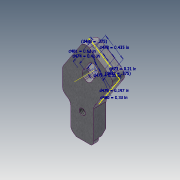
# Autodesk Inventor part: J005520
Saved by Autodesk Inventor 2015 SP1 (Build 190203100, 203)
## iProperties
Created: 2014-10-30
Material: STAINLESS STEEL, 303
Vendor: HHMI: JFRC - ID&F
Document SubType Name: Modeling
Designer: arnoldj
Density: 8 g/cm^3
Mass: 37.2011 g
Surface Area: 34.3864 cm^2
Volume: 4.65014 cm^3
Description: MBS TRAINER CLAMP ARM
Project: P-201804
Appearance: Metal-Steel (Stainless, Brushed)
Part Number: J005520
RuleStatus: InUse
AfterDocSave0: file://Part Number Cleaner
LAB/DEPT: SVOBODA (LAB)
REQUESTING SCIENTIST: SOFRONIEW, NICK
SURFACE ROUGHNESS: 63 Ra
DESIGN DEPARTMENT: HHMI: JRC - ID&F
SPECIAL FINISH: NONE
ALTERED ITEM PART NUMBER: N/A
ALTERED ITEM VENDOR: N/A
ALTERED ITEM DESCRIPTION: N/A
Revision Number: -
Autodesk Inventor part; units mm, degrees
ref_plane "YZ Plane" through (0, 0, 0) normal (1, 0, 0) x (0, 1, 0)
ref_plane "XZ Plane" through (0, 0, 0) normal (0, 1, 0) x (-1, 0, 0)
sketch "Sketch1" plane through (0, 0, 0) normal (0, 0, 1) x (1, 0, 0)
  line L0 (-6, 18.161) -> (6, 18.161)
  line L1 (6, 18.161) -> (6, 0)
  line L2 (6, 0) -> (-6, 0)
  line L3 (-6, 0) -> (-6, 18.161)
  line L4 (0, 70.59) -> (0, -11.765) projected
  line L5 (-14.4746, 0) -> (9.4124, 0) projected
  point P0 (0, 0)
  point P1 (0, 0)
  point P2 (0, 18.161)
  dimension "d0" = 12
  dimension "d1" = 18.161
  constraints: 8 end point, 2 midpoint, 2 parallel, 2 vertical alignment, 1 horizontal, 1 horizontal alignment, 1 perpendicular
  measures "d0" distance of L0.start L0.end
  measures "d1" distance of L2.end L0.start
extrude "Extrusion1" add sketch "Sketch1" along normal blind 2.54
chamfer "Chamfer2" distance 2.54 angle 45 1 edges at (6, 0, 1.27)
chamfer "Chamfer23" distance 3.175 angle 56.5 1 edges at (-6, 0, 1.27) measured on face at (-6, 6.0537, 1.6933)
chamfer "Chamfer5" distance 1.27 angle 45 1 edges at (1.1285, 0, 2.54)
fillet "Fillet4" radius 3.175 4 edges at (3.46, 0, 0.635) (6, 2.54, 1.27) (-6, 3.175, 1.27) (-1.2031, 0, 0.635)
sketch "Sketch32" plane through (0, 0, 0) normal (0, 0, -1) x (-1, 0, 0)
  line L0 (6, 18.161) -> (5.0292, 18.161)
  line L1 (5.0292, 18.161) -> (5.0292, 4.4958)
  line L2 (5.0292, 4.4958) -> (6, 4.4958)
  line L3 (6, 4.4958) -> (6, 18.161)
  line L4 (-6, 18.161) -> (-5.0292, 18.161)
  line L5 (-5.0292, 18.161) -> (-5.0292, 3.8551)
  line L6 (-6, 3.8551) -> (-6, 18.161)
  line L7 (0, -11.765) -> (0, 70.59) projected
  line L8 (-9.4124, 0) -> (14.4746, 0) projected
  line L9 (-6, 3.8551) -> (-5.0292, 3.8551)
  point P0 (0, 0)
  point P1 (-5.0292, 4.4958)
  dimension "d353" = 13.6652
  dimension "d356" = 10.0584
  dimension "d361" = 14.3059
  constraints: 16 end point, 3 horizontal, 3 parallel, 3 point on line, 2 perpendicular, 1 other
  measures "d353" distance of L2.end L0.start
  measures "d356" distance between parallel lines of L5 L1
  measures "d361" distance of L4.end L5.end
sketch "Sketch34" plane through (0, 0, 0) normal (0, 0, 1) x (1, 0, 0)
  line L0 (0, 70.59) -> (0, -11.765) projected
  line L1 (-13.9866, 0) -> (6.4842, 0) projected
  circle A0 centre (0, 5.3848) radius 1.5875
  point P0 (0, 0)
  dimension "d346" = 3.175
  dimension "d347" = 5.3848
  constraints: 1 centre point, 1 point on line
  measures "d346" diameter of A0
  measures "d347" distance from line of L1 A0.centre
extrude "Extrusion25" add sketch "Sketch34" against normal blind 1.143
chamfer "Chamfer24" distance 0.127 angle 45 1 edges at (-1.5875, 5.3848, -1.143)
extrude "Extrusion26" add sketch "Sketch32" along normal blind 3.81
chamfer "Chamfer25" distance 2.54 angle 45 2 edges at (-5.5146, 4.4958, -3.81) (5.5146, 3.8551, -3.81)
fillet "Fillet40" radius 0.254 4 edges at (6, 3.8551, -0.635) (-5.0292, 4.4958, -0.635) (-6, 4.4958, -0.635) (5.0292, 3.8551, -0.635)
sketch "Sketch9" plane through (0, 0, 2.54) normal (0, 0, 1) x (1, 0, 0)
  line L0 (-6, 18.161) -> (6, 18.161) projected
  line L1 (-6, 4.881) -> (-6, 18.161) projected
  line L2 (0, 70.59) -> (0, -11.765) projected
  line L3 (-16.4817, 0) -> (21.4548, 0) projected
  line L4 (6, 19.2992) -> (16.9142, 35.7887)
  line L5 (11.7671, 55.6242) -> (0, 37.846) construction
  line L6 (-10.2361, 29.2838) -> (1.0287, 46.3031)
  line L7 (16.9142, 35.7887) -> (1.0287, 46.3031)
  line L8 (-10.2361, 18.4248) -> (-6, 15.621)
  line L9 (-6, 4.881) -> (-6, 18.161) projected
  line L10 (6, 18.161) -> (6, 3.8551) projected
  line L11 (6, 18.161) -> (6, 3.8551) projected
  line L12 (-6, 15.621) -> (6, 15.621) construction
  line L13 (-6, 18.161) -> (6, 18.161)
  line L14 (6, 18.161) -> (6, 15.621)
  line L15 (-6, 18.161) -> (-6, 15.621)
  line L16 (-10.2361, 18.4248) -> (-10.2361, 29.2838)
  line L17 (6, 18.161) -> (6, 19.2992)
  line L18 (5.0292, 18.161) -> (5.0292, 4.1091) projected
  point P0 (-6.5, 3.8551)
  point P1 (0, 0)
  point P2 (-6, 6.731)
  point P3 (-6, 11.811)
  point P4 (6, 11.811)
  point P5 (6, 6.731)
  dimension "d188" = 19.685
  dimension "d243" = 3.81
  dimension "d244" = 15.24
  dimension "d265" = 2.54
  dimension "d383" = 5.08
  dimension "d384" = 56.5
  dimension "d471" = 7.62
  dimension "d472" = 146.5
  constraints: 22 end point, 3 parallel, 3 point on line, 2 collinear, 2 perpendicular, 2 vertical, 4 other
  measures "d188" distance from line of L0 L5.end
  measures "d243" distance between parallel lines of L5 L6
  measures "d244" distance between parallel lines of L5 L4
  measures "d265" distance from line of L0 L8.end
  measures "d383" distance of L8.start L8.end
  measures "d384" angle to the sketch y axis of L8
  measures "d471" distance from line of L5.end L7
  measures "d472" angle of L4 L17
extrude "Extrusion6-Main Body" add sketch "Sketch9" against normal blind 6.35
sketch "Sketch37" plane through (0, 0, -3.81) normal (0, 0, -1) x (-1, 0, 0)
  line L0 (-16.9142, 35.7887) -> (-1.0287, 46.3031) projected
  line L1 (-6.8533, 42.4478) -> (-13.7371, 37.8916)
  line L2 (-13.7371, 37.8916) -> (10.2361, 1.672)
  line L3 (10.2361, 29.2838) -> (10.2361, 18.4248) projected
  line L4 (10.2361, 16.6284) -> (10.2361, 1.672)
  line L5 (10.2361, 29.2838) -> (10.2361, 18.4248) projected
  line L6 (10.2361, 16.6284) -> (-6.8533, 42.4478)
  line L7 (-16.9142, 35.7887) -> (-1.0287, 46.3031) projected
  line L8 (-6, 19.2992) -> (-16.9142, 35.7887) projected
  point P0 (0, 0)
  point P1 (-7.016, 38.7359)
  dimension "d420" = 8.255
  dimension "d465" = 3.81
  constraints: 8 end point, 4 point on line, 2 perpendicular, 1 collinear, 1 other
  measures "d420" distance between parallel lines of L2 L6
extrude "Extrusion29" [suppressed]
sketch "Sketch38" plane through (0, 0, -6.35) normal (0, 0, -1) x (-1, 0, 0)
  line L0 (-8.8086, 55.8253) -> (11.0622, 25.8039) construction
  line L1 (-3.2486, 59.5053) -> (11.0622, 37.884) construction
  line L2 (7.204, 31.633) -> (12.7639, 35.313) construction
  line L3 (-3.3104, 47.5185) -> (2.2495, 51.1985) construction
  line L4 (0.1944, 42.2233) -> (5.7543, 45.9034) construction
  line L5 (3.6992, 36.9282) -> (9.2591, 40.6082) construction
  circle A0 centre (-3.3104, 47.5185) radius 2.5 construction
  circle A1 centre (7.204, 31.633) radius 2.5 construction
  line L6 (-4.6903, 49.6032) -> (-5.9372, 48.7779) construction
  line L7 (-12.2504, 53.5472) -> (11.0622, 18.3257) projected
  line L8 (11.0622, 33.2821) -> (-5.3667, 58.1034) projected
  line L9 (-5.3667, 58.1034) -> (-12.2504, 53.5472) projected
  line L10 (11.0622, 18.3257) -> (11.0622, 33.2821) projected
  line L11 (-6.8152, 52.8137) -> (-1.2553, 56.4937) construction
  line L12 (-3.2486, 59.5053) -> (11.0622, 37.884) construction
  line L13 (-5.3667, 58.1034) -> (-3.2486, 59.5053) projected
  line L14 (-21.0658, 0) -> (18.4022, 0) projected
  point P0 (0, 0)
  point P1 (-3.5598, 58.825)
  dimension "d415" = 5
  dimension "d407" = 6.35
  dimension "d410" = 6.35
  dimension "d411" = 6.35
  dimension "d412" = 9.9615
  dimension "d413" = 6.9903
  dimension "d416" = 5
  dimension "d421" = 8.255
  dimension "d422" = 4.1275
  dimension "d427" = 6.35
  dimension "d461" = 19.6903
  dimension "d464" = 42.2233
  constraints: 14 end point, 7 point on line, 2 coincident, 2 midpoint, 1 centre point, 1 parallel, 1 perpendicular, 15 other
  measures "d407" distance between parallel lines of L3 L4
  measures "d410" distance between parallel lines of L4 L5
  measures "d411" distance between parallel lines of L2 L5
  measures "d412" distance from line of L0.start L3
  measures "d413" distance from line of L0.end L2
  measures "d416" diameter of A1
  measures "d421" distance between parallel lines of L7 L8
  measures "d422" distance between parallel lines of L7 L0
  measures "d427" distance from line of L3 L11.start
  measures "d461" distance from line of L0.end L4
  measures "d464" distance from line of L4.start L14
hole "Hole3" [suppressed]
fillet "Fillet46" [suppressed]
fillet "Fillet47" [suppressed]
fillet "Fillet48" [suppressed]
sketch "Sketch39" plane through (0, 0, -3.81) normal (0, 0, -1) x (-1, 0, 0)
  line L0 (5.0292, 18.161) -> (-5.0292, 18.161)
  line L1 (5.0292, 18.161) -> (-5.0292, 18.161)
  line L2 (-5.0292, 18.161) -> (-5.0292, 23.876)
  line L3 (-5.0292, 23.876) -> (5.0292, 23.876)
  line L4 (5.0292, 23.876) -> (5.0292, 18.161)
  line L5 (5.0292, 18.161) -> (-5.0292, 18.161)
  line L6 (0, -9.2606) -> (0, 55.5637) projected
  line L7 (-22.3442, 0) -> (15.6662, 0) projected
  point P0 (0, 0)
  dimension "d429" = 5.715
  dimension "d433" = 18.161
  dimension "d434" = 5.0292
  dimension "d435" = 10.0584
  constraints: 12 end point, 3 equal length, 1 perpendicular
  measures "d429" distance of L3.end L0.start
  measures "d433" distance between parallel lines of L7 L0
  measures "d434" distance between parallel lines of L6 L4
  measures "d435" distance of L2.end L3.end
extrude "Extrusion30" cut sketch "Sketch39" against normal blind 3.81
sketch "Sketch41" plane through (0, 0, 0) normal (0, 0, -1) x (-1, 0, 0)
  line L0 (5.0292, 23.876) -> (-5.0292, 23.876)
  line L1 (-5.0292, 23.876) -> (-5.0292, 10.795)
  line L2 (-5.0292, 10.795) -> (5.0292, 10.795)
  line L3 (5.0292, 10.795) -> (5.0292, 23.876)
  line L4 (-5.0292, 23.876) -> (-5.0292, 4.1091) projected
  point P0 (0, 0)
  dimension "d439" = 10.795
  constraints: 8 end point, 2 parallel, 2 perpendicular
  measures "d439" distance from line of L2 point (0, 0)
extrude "Extrusion31" add sketch "Sketch41" along normal blind 0.635
fillet "Fillet49" radius 1.651 4 edges at (-5.0292, 23.876, -2.2225) (5.0292, 23.876, -2.2225) (-5.0292, 10.795, -0.3175) (5.0292, 10.795, -0.3175)
sketch "Sketch42" plane through (0, 0, -3.81) normal (0, 0, -1) x (-1, 0, 0)
  point P0 (0, 0)
sketch "Sketch43" plane through (0, 0, -3.81) normal (0, 0, -1) x (-1, 0, 0)
  line L0 (0, -9.2606) -> (0, 55.5637) projected
  line L1 (-22.3442, 0) -> (15.6662, 0) projected
  line L2 (-3.3782, 23.876) -> (3.3782, 23.876) projected
  point P0 (0, 0)
  point P1 (0, 13.97)
  dimension "d450" = 13.97
  dimension "d458" = 9.906
  dimension "d459" = 23.876
  constraints: 1 point on line
  measures "d450" distance from line of L1 point (0, 13.97)
  measures "d458" distance from line of point (0, 13.97) L2
  measures "d459" distance from line of point (0, 0) L2
hole "Hole5" at (0, 13.97, -3.81) direction (0, 0, 1) diameter 3.2512 end through all
sketch "Sketch45" plane through (0, 0, 0) normal (0, 0, 1) x (1, 0, 0)
  line L0 (16.9142, 35.7887) -> (1.0287, 46.3031) projected
  line L1 (1.0287, 46.3031) -> (-10.2361, 29.2838) projected
  line L2 (6, 19.2992) -> (16.9142, 35.7887) projected
  line L3 (8.9714, 41.0459) -> (-7.2913, 16.4757) construction
  line L4 (-10.2361, 18.4248) -> (-6, 15.621) construction
  line L5 (3.4147, 27.8186) -> (9.1626, 36.5027)
  line L6 (9.1626, 36.5027) -> (4.7147, 39.4467)
  line L7 (4.7147, 39.4467) -> (-1.0332, 30.7626)
  line L8 (-1.0332, 30.7626) -> (3.4147, 27.8186)
  line L9 (3.4147, 27.8186) -> (4.7147, 39.4467) construction
  line L10 (9.1626, 36.5027) -> (-1.0332, 30.7626) construction
  line L11 (4.3956, 24.1234) -> (12.9474, 37.0436)
  line L12 (12.9474, 37.0436) -> (3.7338, 43.1419)
  line L13 (3.7338, 43.1419) -> (-4.818, 30.2217)
  line L14 (-4.818, 30.2217) -> (4.3956, 24.1234)
  line L15 (4.3956, 24.1234) -> (3.7338, 43.1419) construction
  line L16 (12.9474, 37.0436) -> (-4.818, 30.2217) construction
  circle A0 centre (5.4684, 35.7534) radius 2.5019 construction
  circle A1 centre (5.4684, 35.7534) radius 4.191 construction
  point P0 (0, 0)
  point P1 (4.0647, 33.6326)
  point P2 (4.0647, 33.6326)
  dimension "d473" = 5.334
  dimension "d474" = 10.414
  dimension "d475" = 8.89
  dimension "d478" = 11.049
  dimension "d479" = 5.0038
  dimension "d480" = 8.382
  dimension "d481" = 15.494
  dimension "d487" = 9.525
  dimension "d488" = 9.525
  constraints: 26 end point, 7 parallel, 5 midpoint, 3 point on line, 2 centre point, 2 coincident, 2 perpendicular
  measures "d473" distance of L5.end L6.end
  measures "d474" distance of L6.end L7.end
  measures "d475" distance from line of L0 point (4.065, 33.633)
  measures "d478" distance of L11.end L12.end
  measures "d479" diameter of A0
  measures "d480" diameter of A1
  measures "d481" distance of L12.end L13.end
  measures "d487" distance between parallel lines of L2 L3
  measures "d488" distance between parallel lines of L3 L1
extrude "Extrusion33" cut sketch "Sketch45" along normal mid plane 25.4 contours L8 L7 L6 L5
sketch "Sketch47" plane through (0, 0, -3.81) normal (0, 0, -1) x (-1, 0, 0)
  line L0 (-12.9474, 37.0436) -> (-3.7338, 43.1419) projected
  line L1 (-3.7338, 43.1419) -> (4.818, 30.2217) projected
  line L2 (-4.3956, 24.1234) -> (-12.9474, 37.0436) projected
  line L3 (4.818, 30.2217) -> (-4.3956, 24.1234) projected
  point P0 (0, 0)
extrude "Extrusion34" cut sketch "Sketch47" against normal blind 3.175
fillet "Fillet50" radius 2.3813 4 edges at (3.4147, 27.8186, 0.9525) (9.1626, 36.5027, 0.9525) (4.7147, 39.4467, 0.9525) (-1.0332, 30.7626, 0.9525)
fillet "Fillet51" radius 3.175 4 edges at (4.3956, 24.1234, -2.2225) (-4.818, 30.2217, -2.2225) (12.9474, 37.0436, -2.2225) (3.7338, 43.1419, -2.2225)
fillet "Fillet52" radius 3.175 6 edges at (6, 19.2992, -0.635) (16.9142, 35.7887, -0.635) (1.0287, 46.3031, -0.635) (-10.2361, 29.2838, -0.635) (-10.2361, 18.4248, -0.635) (-6, 15.621, -0.635)
body "Solid1"
